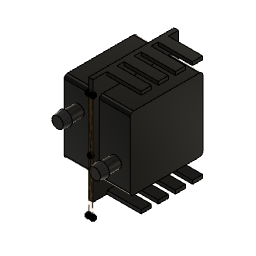
Amphenol Pressure Sensor (Autodesk Fusion 360 design; units mm, degrees)
Autodesk Fusion 360 part; units mm, degrees
ref_plane "WorkPlane1" through (-0.72, 10, 0) normal (-1, 0, 0) x (0, -1, 0)
sketch "Sketch1" plane through (-0.72, 30, 34.5) normal (-1, 0, 0) x (0, 1, 0)
  line L0 (8.3928, -23.0007) -> (-4.3072, -23.0007)
  line L1 (-4.3072, -23.0007) -> (-4.3072, -7.2527)
  line L2 (-4.3072, -7.2527) -> (8.3928, -7.2527)
  line L3 (8.3928, -7.2527) -> (8.3928, -23.0007)
  dimension "d49" = 12.7
  dimension "d50" = 15.748
  constraint horizontal L0
  constraint vertical L1
  constraint horizontal L2
  constraint vertical L3
  measures "d49" distance of L0.start L0.end
  measures "d50" distance of L0.start L2.end
extrude "Extrude1" add sketch "Sketch1" against normal blind 0.64
sketch "Sketch2" plane through (-0.72, 0, 0) normal (-1, 0, 0) x (0, -1, 0)
  line L0 (-38.3928, 41.7527) -> (-25.6928, 41.7527)
  line L1 (-25.6928, 41.7527) -> (-25.6928, 57.5007)
  line L2 (-25.6928, 57.5007) -> (-38.3928, 57.5007)
  line L3 (-38.3928, 57.5007) -> (-38.3928, 41.7527)
  line L4 (-38.3928, 57.5007) -> (-25.6928, 41.7527) construction
  line L5 (-25.6928, 57.5007) -> (-38.3928, 41.7527) construction
  line L6 (-37.4428, 55.0267) -> (-26.6428, 55.0267)
  line L7 (-26.6428, 55.0267) -> (-26.6428, 44.2267)
  line L8 (-26.6428, 44.2267) -> (-37.4428, 44.2267)
  line L9 (-37.4428, 44.2267) -> (-37.4428, 55.0267)
  line L10 (-37.4428, 55.0267) -> (-26.6428, 44.2267) construction
  line L11 (-26.6428, 55.0267) -> (-37.4428, 44.2267) construction
  point P0 (-32.0428, 49.6267)
  dimension "d53" = 10.8
  dimension "d54" = 10.8
  constraint coincident L2.end L3.start
  constraint coincident L0.end L1.start
  constraint coincident L1.end L2.start
  constraint coincident L0.start L3.end
  constraint perpendicular L6 L7
  constraint parallel L6 L8
  constraint parallel L7 L9
  constraint horizontal L6
  constraint coincident L10 P0
  constraint coincident L11 P0
  constraint midpoint L5 P0
  measures "d53" distance of L7.end L8.end
  measures "d54" distance of L6.end L7.end
extrude "Extrude2" add sketch "Sketch2" along normal blind 4.572 contours L6 L7 L8 L9
sketch "Sketch3" plane through (0, 26.6428, 0) normal (0, -1, 0) x (1, 0, 0)
  line L0 (-0.72, 44.2267) -> (-0.72, 55.0267)
  line L1 (-0.72, 55.0267) -> (-5.292, 55.0267)
  line L2 (-5.292, 55.0267) -> (-5.292, 44.2267)
  line L3 (-5.292, 44.2267) -> (-0.72, 44.2267)
  circle A0 centre (-3.16, 51.5527) radius 0.84
  line L4 (-0.72, 57.5007) -> (-0.72, 41.7527)
  point P0 (-0.72, 41.7527)
  dimension "d57" = 1.68
  dimension "d59" = 9.8
  dimension "d60" = 2.44
  measures "d57" diameter of A0
  measures "d59" vertical distance of A0.centre P0
  measures "d60" distance of A0.centre L4
extrude "Extrude3" add sketch "Sketch3" along normal blind 3.11 contours A0
sketch "Sketch4" plane through (0, 23.5328, 0) normal (0, -1, 0) x (1, 0, 0)
  circle A0 centre (-3.16, 51.5527) radius 0.84
extrude "Extrude4" add sketch "Sketch4" against normal blind 1.14 draft 10
fillet "Fillet1" radius 0.5 4 edges at (-3.006, 26.6428, 55.0267) (-3.006, 37.4428, 55.0267) (-3.006, 37.4428, 44.2267) (-3.006, 26.6428, 44.2267)
sketch "Sketch5" plane through (0, 25.6928, 0) normal (0, -1, 0) x (1, 0, 0)
  line L0 (-0.72, 57.5007) -> (-0.72, 41.7527)
  line L1 (-0.72, 41.7527) -> (-0.08, 41.7527)
  line L2 (-0.08, 41.7527) -> (-0.08, 57.5007)
  line L3 (-0.08, 57.5007) -> (-0.72, 57.5007)
  line L4 (-0.72, 41.7527) -> (-0.08, 57.5007) construction
  line L5 (-0.72, 57.5007) -> (-0.08, 41.7527) construction
  point P0 (-0.4, 49.6267)
  constraint coincident L0.end L1.start
  constraint coincident L2.end L3.start
  constraint coincident L0.start L3.end
  constraint coincident L1.end L2.start
  constraint midpoint L5 P0
pattern_circular "C-Pattern1" count 2 over 360 about axis through (-0.4, 41.4408, 49.6267) along (0, -1, 0) of 13 faces at (-3.0364, 26.6428, 46.7228) (-2.2623, 24.4194, 51.985) (-3.3191, 23.5328, 52.1899) (-2.6697, 25.9861, 52.2347) (-5.292, 30.4094, 51.4267) (-2.244, 26.6569, 54.6445) (-2.244, 26.6569, 44.6088) (-2.244, 30.4094, 44.2267) (-4.1301, 24.6728, 51.5009) (-2.244, 37.0606, 44.2407) (-2.244, 37.4428, 47.9933) (-2.244, 37.0606, 55.0126) (-2.244, 33.6761, 55.0267)
sketch "Sketch6" plane through (-0.72, 0, 0) normal (-1, 0, 0) x (0, -1, 0)
  line L0 (-37.4428, 44.7267) -> (-37.4428, 54.5267)
  arc A0 (-36.9428, 55.0267) -> (-37.4428, 54.5267) centre (-36.9428, 54.5267) ccw
  line L1 (-36.9428, 55.0267) -> (-27.1428, 55.0267)
  arc A1 (-26.6428, 54.5267) -> (-27.1428, 55.0267) centre (-27.1428, 54.5267) ccw
  line L2 (-26.6428, 54.5267) -> (-26.6428, 44.7267)
  arc A2 (-27.1428, 44.2267) -> (-26.6428, 44.7267) centre (-27.1428, 44.7267) ccw
  line L3 (-27.1428, 44.2267) -> (-36.9428, 44.2267)
  arc A3 (-37.4428, 44.7267) -> (-36.9428, 44.2267) centre (-36.9428, 44.7267) ccw
  line L4 (-38.3928, 41.7527) -> (-25.6928, 41.7527)
  line L5 (-25.6928, 41.7527) -> (-25.6928, 57.5007)
  line L6 (-25.6928, 57.5007) -> (-38.3928, 57.5007)
  line L7 (-38.3928, 57.5007) -> (-38.3928, 41.7527)
  line L8 (-36.8928, 41.7527) -> (-35.3928, 41.7527)
  line L9 (-35.3928, 41.7527) -> (-35.3928, 42.2527)
  line L10 (-35.3928, 42.2527) -> (-36.8928, 42.2527)
  line L11 (-36.8928, 42.2527) -> (-36.8928, 41.7527)
  line L12 (-32.8528, 42.2527) -> (-34.3528, 42.2527)
  line L13 (-34.3528, 42.2527) -> (-34.3528, 41.7527)
  line L14 (-34.3528, 41.7527) -> (-32.8528, 41.7527)
  line L15 (-32.8528, 41.7527) -> (-32.8528, 42.2527)
  line L16 (-30.3128, 42.2527) -> (-31.8128, 42.2527)
  line L17 (-31.8128, 42.2527) -> (-31.8128, 41.7527)
  line L18 (-31.8128, 41.7527) -> (-30.3128, 41.7527)
  line L19 (-30.3128, 41.7527) -> (-30.3128, 42.2527)
  line L20 (-27.7728, 42.2527) -> (-29.2728, 42.2527)
  line L21 (-29.2728, 42.2527) -> (-29.2728, 41.7527)
  line L22 (-29.2728, 41.7527) -> (-27.7728, 41.7527)
  line L23 (-27.7728, 41.7527) -> (-27.7728, 42.2527)
  line L24 (-35.3928, 57.5027) -> (-36.8928, 57.5027)
  line L25 (-36.8928, 57.5027) -> (-36.8928, 57.0027)
  line L26 (-36.8928, 57.0027) -> (-35.3928, 57.0027)
  line L27 (-35.3928, 57.0027) -> (-35.3928, 57.5027)
  line L28 (-32.8528, 57.5027) -> (-34.3528, 57.5027)
  line L29 (-34.3528, 57.5027) -> (-34.3528, 57.0027)
  line L30 (-34.3528, 57.0027) -> (-32.8528, 57.0027)
  line L31 (-32.8528, 57.0027) -> (-32.8528, 57.5027)
  line L32 (-30.3128, 57.5027) -> (-31.8128, 57.5027)
  line L33 (-31.8128, 57.5027) -> (-31.8128, 57.0027)
  line L34 (-31.8128, 57.0027) -> (-30.3128, 57.0027)
  line L35 (-30.3128, 57.0027) -> (-30.3128, 57.5027)
  line L36 (-27.7728, 57.5027) -> (-29.2728, 57.5027)
  line L37 (-29.2728, 57.5027) -> (-29.2728, 57.0027)
  line L38 (-29.2728, 57.0027) -> (-27.7728, 57.0027)
  line L39 (-27.7728, 57.0027) -> (-27.7728, 57.5027)
  dimension "d68" = 1.5
  dimension "d69" = 0.5
  dimension "d70" = 1.5
  dimension "d73" = 2.54
  dimension "d74" = 15.25
  constraint horizontal L8
  constraint vertical L9
  constraint horizontal L10
  constraint vertical L11
  constraint coincident L4 L8.start
  measures "d68" distance of L8.start L8.end
  measures "d69" distance of L8.start L10.end
  measures "d70" distance of L7 L10.end
extrude "Extrude5" add sketch "Sketch6" against normal blind 5.72 contours L4 L8 L9 L10 L11 | L6 L24 L25 L26 L27 | L4 L12 L13 L14 L15 | L6 L28 L29 L30 L31 | L4 L16 L17 L18 L19 | L6 L32 L33 L34 L35 | L4 L20 L21 L22 L23 | L6 L36 L37 L38 L39
move_body "Move1" bodies 1 to x (1, 0, 0) y (0, 1, 0) z (0, 0, 1) at (0, 0, 2)
equation "d60 = ( 4.88 / 2 ) * 1 mm"
